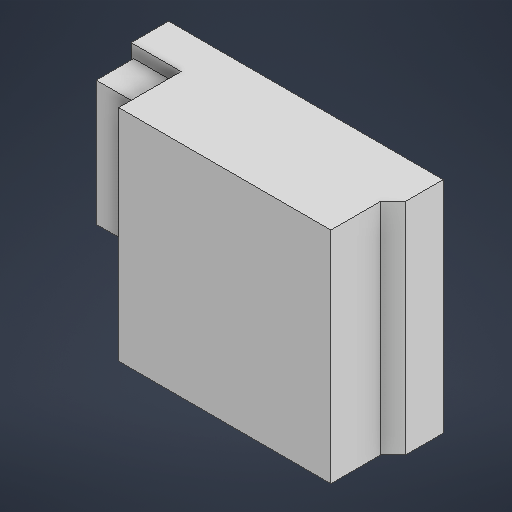
# Autodesk Inventor part: PowerSupply
Saved by Autodesk Inventor 2026.2 (Build 302298000, 298)
## iProperties
Created: 2026-01-21
Part Number: PowerSupply
Material: Generic
Document SubType Name: Modeling
Designer: User
Density: 1 g/cm^3
Appearance: Default
Author: User
Autodesk Inventor part; units mm, degrees
ref_plane "YZ Plane" through (0, 0, 0) normal (1, 0, 0) x (0, 1, 0)
ref_plane "XZ Plane" through (0, 0, 0) normal (0, 1, 0) x (-1, 0, 0)
ref_plane "XY Plane" through (0, 0, 0) normal (0, 0, 1) x (1, 0, 0)
sketch "Sketch2" plane through (0, 0, 0) normal (0, 1, 0) x (-1, 0, 0)
  line L0 (0, 0) -> (85, 0)
  line L1 (85, 0) -> (85, -25)
  line L2 (85, -25) -> (0, -25)
  line L3 (0, -25) -> (0, 0)
  line L4 (-5, -25) -> (105, -25)
  line L5 (105, -25) -> (105, -40)
  line L6 (105, -40) -> (-5, -40)
  line L7 (-5, -40) -> (-5, -25)
  line L8 (-5, -25) -> (0, -20)
  dimension "d4" = 85
  dimension "d5" = 25
  dimension "d6" = 110
  dimension "d7" = 5
  dimension "d8" = 15
  dimension "d9" = 45
  constraints: 18 end point, 4 parallel, 2 horizontal, 2 perpendicular, 2 point on line
  measures "d4" distance of L0.start L0.end
  measures "d5" distance of L0.end L1.end
  measures "d6" distance of L5.end L6.end
  measures "d7" distance between parallel lines of L3 L7
  measures "d8" distance of L4.end L5.end
  measures "d9" angle of L4 L8
extrude "Extrusion2" add sketch "Sketch2" along normal blind 88
sketch "Sketch3" plane through (-105, 0, -25) normal (0, 0, 1) x (1, 0, 0)
  line L0 (20, 0) -> (20, 88) projected
  line L1 (20, 83) -> (1, 83)
  line L2 (1, 83) -> (1, 33)
  line L3 (1, 33) -> (20, 33)
  line L4 (20, 33) -> (20, 83)
  line L5 (0, 88) -> (20, 88) projected
  point P0 (105, 0)
  point P1 (20, 33)
  dimension "d12" = 50
  dimension "d13" = 19
  dimension "d14" = 5
  constraints: 8 end point, 2 parallel, 1 horizontal, 1 perpendicular, 1 point on line
  measures "d12" distance of L1.end L2.end
  measures "d13" distance of L1.start L1.end
  measures "d14" distance between parallel lines of L5 L1
extrude "Extrusion3" add sketch "Sketch3" along normal blind 15
sketch "Sketch4" plane through (-104, 33, -25) normal (-1, 0, 0) x (0, 0, 1)
  line L0 (6, 7.5) -> (11, 7.5)
  line L1 (11, 7.5) -> (11, 2.5)
  line L2 (11, 2.5) -> (6, 2.5)
  line L3 (6, 2.5) -> (6, 7.5)
  line L4 (0, -33) -> (0, 55) projected
  line L5 (0, 0) -> (15, 0) projected
  line L6 (6, 17.5) -> (11, 17.5)
  line L7 (11, 17.5) -> (11, 12.5)
  line L8 (6, 12.5) -> (6, 17.5)
  line L9 (11, 12.5) -> (6, 12.5)
  line L10 (6, 27.5) -> (11, 27.5)
  line L11 (11, 27.5) -> (11, 22.5)
  line L12 (6, 22.5) -> (6, 27.5)
  line L13 (11, 22.5) -> (6, 22.5)
  line L14 (6, 37.5) -> (11, 37.5)
  line L15 (11, 37.5) -> (11, 32.5)
  line L16 (6, 32.5) -> (6, 37.5)
  line L17 (11, 32.5) -> (6, 32.5)
  line L18 (6, 47.5) -> (11, 47.5)
  line L19 (11, 47.5) -> (11, 42.5)
  line L20 (6, 42.5) -> (6, 47.5)
  line L21 (11, 42.5) -> (6, 42.5)
  point P0 (25, -33)
  point P1 (6, 5)
  point P2 (7.5, 0)
  point P3 (8.5, 2.5)
  point P4 (6, 15)
  point P5 (8.5, 12.5)
  point P6 (6, 25)
  point P7 (8.5, 22.5)
  point P8 (6, 35)
  point P9 (8.5, 32.5)
  point P10 (6, 45)
  point P11 (8.5, 42.5)
  dimension "d17" = 6
  dimension "d18" = 5
  dimension "d19" = 2.5
  dimension "d20" = 5
  dimension "d23" = 10
  constraints: 40 end point, 3 midpoint, 2 parallel, 1 horizontal, 1 perpendicular, 1 vertical, 40 other
  measures "d17" distance from line of L4 point (6, 5)
  measures "d18" distance of L0.start L0.end
  measures "d19" vertical distance of point (7.5, 0) point (8.5, 2.5)
  measures "d20" distance of L0.end L1.end
  measures "d23" distance of L0.start L6.start
extrude "Extrusion4" cut sketch "Sketch4" against normal blind 10
body "Solid2"
